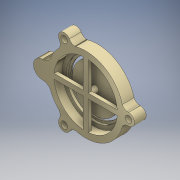
# Autodesk Inventor part: ET3
Saved by Autodesk Inventor 2016 (Build 200138000, 138)
## iProperties
Created: 2016-03-19
Part Number: ET3
Material: Genérico
Document SubType Name: Modeling
Designer: Usuario1
Density: 1 g/cm^3
Appearance: Valor por defecto
Author: Usuario1
Autodesk Inventor part; units mm, degrees
ref_plane "YZ Plane" through (0, 0, 0) normal (1, 0, 0) x (0, 1, 0)
ref_plane "XZ Plane" through (0, 0, 0) normal (0, 1, 0) x (-1, 0, 0)
ref_plane "XY Plane" through (0, 0, 0) normal (0, 0, 1) x (1, 0, 0)
sketch "Boceto1" plane through (0, 0, 0) normal (0, 1, 0) x (-1, 0, 0)
  circle A0 centre (-2.5469, -0.001) radius 0.2
  arc A1 (2.5775, -0.5336) -> (2.5774, 0.5316) centre (2.5775, -0.001) ccw
  circle A2 centre (2.5775, -0.001) radius 0.4
  arc A3 (2.5775, -0.5336) -> (2.1206, -0.7589) centre (2.5776, -1.11) ccw
  arc A4 (2.1204, 0.7569) -> (2.5774, 0.5316) centre (2.5774, 1.108) ccw
  arc A5 (-2.5469, 0.349) -> (-2.1734, 0.574) centre (-2.5174, 0.7225) ccw
  arc A6 (-2.1734, -0.576) -> (-2.5469, -0.351) centre (-2.5174, -0.7245) ccw
  arc A7 (-2.5469, 0.349) -> (-2.5469, -0.351) centre (-2.5469, -0.001) ccw
  circle A8 centre (1.2763, 2.2063) radius 0.2
  arc A9 (1.5794, 2.0313) -> (1.5874, 1.5954) centre (1.888, 1.819) ccw
  arc A10 (0.5916, 2.1703) -> (0.9731, 2.3813) centre (0.6349, 2.5425) ccw
  arc A11 (1.5794, 2.0313) -> (0.9731, 2.3813) centre (1.2763, 2.2063) ccw
  circle A12 centre (1.2764, -2.2083) radius 0.2
  arc A13 (0.9733, -2.3833) -> (0.5918, -2.1723) centre (0.6351, -2.5444) ccw
  arc A14 (1.5879, -1.5974) -> (1.5796, -2.0333) centre (1.8883, -1.8211) ccw
  arc A15 (0.9733, -2.3833) -> (1.5796, -2.0333) centre (1.2764, -2.2083) ccw
  circle A16 centre (0.0019, -0.001) radius 1.8825
  arc A17 (-2.1734, -0.576) -> (0.5918, -2.1723) centre (0.0019, -0.001) ccw
  arc A18 (0.5916, 2.1703) -> (-2.1734, 0.574) centre (0.0019, -0.001) ccw
  arc A19 (2.1204, 0.7569) -> (1.5874, 1.5954) centre (0.0019, -0.001) ccw
  arc A20 (1.5879, -1.5974) -> (2.1206, -0.7589) centre (0, 0) ccw
  constraints: 36 point on circle, 21 centre point
extrude "Extrusión1" add sketch "Boceto1" along normal blind 0.7
sketch "Boceto2" plane through (0, 0, 0) normal (0, 1, 0) x (-1, 0, 0)
  circle A0 centre (-2.5469, -0.001) radius 0.2
  arc A1 (2.5775, -0.5336) -> (2.5774, 0.5316) centre (2.5775, -0.001) ccw
  circle A2 centre (2.5775, -0.001) radius 0.4
  arc A3 (2.5775, -0.5336) -> (2.1206, -0.7589) centre (2.5776, -1.11) ccw
  arc A4 (2.1204, 0.7569) -> (2.5774, 0.5316) centre (2.5774, 1.108) ccw
  arc A5 (-2.5469, 0.349) -> (-2.1734, 0.574) centre (-2.5174, 0.7225) ccw
  arc A6 (-2.1734, -0.576) -> (-2.5469, -0.351) centre (-2.5174, -0.7245) ccw
  arc A7 (-2.5469, 0.349) -> (-2.5469, -0.351) centre (-2.5469, -0.001) ccw
  circle A8 centre (1.2763, 2.2063) radius 0.2
  arc A9 (1.5794, 2.0313) -> (1.5874, 1.5954) centre (1.888, 1.819) ccw
  arc A10 (0.5916, 2.1703) -> (0.9731, 2.3813) centre (0.6349, 2.5425) ccw
  arc A11 (1.5794, 2.0313) -> (0.9731, 2.3813) centre (1.2763, 2.2063) ccw
  circle A12 centre (1.2764, -2.2083) radius 0.2
  arc A13 (0.9733, -2.3833) -> (0.5918, -2.1723) centre (0.6351, -2.5444) ccw
  arc A14 (1.5879, -1.5974) -> (1.5796, -2.0333) centre (1.8883, -1.8211) ccw
  arc A15 (0.9733, -2.3833) -> (1.5796, -2.0333) centre (1.2764, -2.2083) ccw
  circle A16 centre (0.0019, -0.001) radius 1.8825
  arc A17 (-2.1734, -0.576) -> (0.5918, -2.1723) centre (0.0019, -0.001) ccw
  arc A18 (0.5916, 2.1703) -> (-2.1734, 0.574) centre (0.0019, -0.001) ccw
  arc A19 (2.1204, 0.7569) -> (1.5874, 1.5954) centre (0.0019, -0.001) ccw
  arc A20 (1.5879, -1.5974) -> (2.1206, -0.7589) centre (0, 0) ccw
  point P0 (0, 0)
  constraints: 36 point on circle, 21 centre point
extrude "Extrusión2" add sketch "Boceto2" along normal blind 0.5 contours A2
sketch "Boceto3" plane through (0, 0.7, 0) normal (0, 1, 0) x (1, 0, 0)
  circle A0 centre (-0.0019, 0.001) radius 1.8825 projected
  point P0 (0, 0)
extrude "Extrusión3" add sketch "Boceto3" against normal blind 0.06
sketch "Boceto4" plane through (-0.0019, 0.64, -0.001) normal (0, -1, 0) x (1, 0, 0)
  circle A0 centre (0.0019, 0.001) radius 1.65
  circle A1 centre (0, 0) radius 1.8825 projected
  dimension "d6" = 3.3
  constraints: 1 centre point, 1 coincident
  measures "d6" diameter of A0
extrude "Extrusión4" add sketch "Boceto4" along normal blind 0.15
sketch "Boceto5" plane through (0, 0.7, 0) normal (0, 1, 0) x (1, 0, 0)
  circle A0 centre (0, 0) radius 1.525
  circle A1 centre (0, 0) radius 1.375
  dimension "d9" = 3.05
  dimension "d11" = 2.75
  constraints: 2 centre point, 1 coincident
  measures "d9" diameter of A0
  measures "d11" diameter of A1
extrude "Extrusión5" cut sketch "Boceto5" against normal blind 0.1
sketch "Boceto6" plane through (0, 0.64, 0) normal (0, -1, 0) x (1, 0, 0)
  circle A0 centre (0, 0) radius 0.2
  dimension "d14" = 0.4
  constraints: 1 centre point, 1 coincident
  measures "d14" diameter of A0
extrude "Extrusión6" add sketch "Boceto6" along normal blind 0.64
sketch "Boceto7" plane through (0, 0, 0) normal (0, -1, 0) x (1, 0, 0)
  circle A0 centre (-0.0019, -0.001) radius 1.8825 projected
  line L0 (-0.1519, -1.8835) -> (-0.1519, 1.8815)
  line L1 (1.8726, 0.15) -> (-1.8844, 0.15)
  line L2 (1.8726, -0.15) -> (-1.8844, -0.15)
  line L3 (0.1481, -1.8835) -> (0.1481, 1.8815)
  line L4 (1.8726, -0.15) -> (1.9479, -0.15)
  line L5 (1.9479, -0.15) -> (1.9479, 0.15)
  line L6 (1.9479, 0.15) -> (1.8726, 0.15)
  line L7 (-0.1519, -1.8835) -> (0.1481, -1.8835)
  line L8 (-1.8844, -0.15) -> (-1.8844, 0.15)
  line L9 (0.1481, 1.8815) -> (-0.1519, 1.8815)
  point P0 (0, 0)
  constraints: 20 end point, 3 perpendicular, 1 collinear, 1 horizontal, 1 parallel
extrude "Extrusión7" add sketch "Boceto7" against normal blind 0.2 contours A0 L2 L3 L1 | A0 L6 L5 L4 | L3 L1 L0 A0 | A0 L9 L3 | L3 L2 L0 L1 | L3 L7 A0 | A0 L0 L2 L3 | A0 L0 L9 | L0 L2 A0 L1 | L7 L0 A0 | A0 L8 L1 | L2 L8 A0
sketch "Boceto8" plane through (0, 0.7, 0) normal (0, 1, 0) x (1, 0, 0)
  circle A0 centre (0, 0) radius 1.8875
  circle A1 centre (0, 0) radius 1.525 projected
  circle A2 centre (0, 0) radius 1.375 projected
  dimension "d23" = 3.775
  constraints: 1 centre point, 1 coincident
  measures "d23" diameter of A0
extrude "Extrusión8" add sketch "Boceto8" along normal blind 0.02
sketch "Boceto9" plane through (0, 0.64, 0) normal (0, -1, 0) x (1, 0, 0)
  circle A0 centre (0, 0) radius 0.2 projected
  circle A1 centre (0, 0) radius 1.375 projected
extrude "Extrusión9" add sketch "Boceto9" along normal blind 0.07
